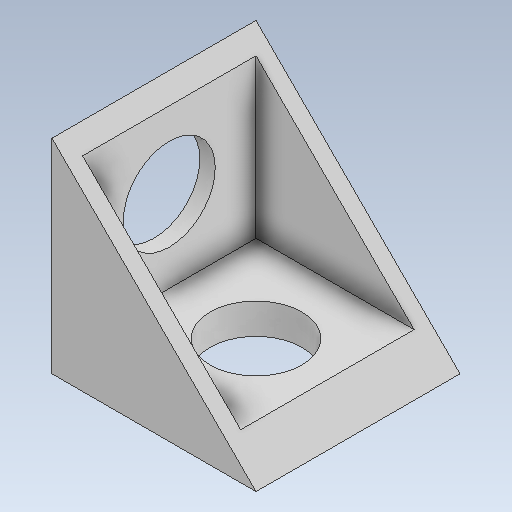
# Autodesk Inventor part: corner bracket
Saved by Autodesk Inventor 2023 (Build 270158000, 158)
## iProperties
Created: 2023-01-21
Part Number: corner bracket
Material: Generic
Document SubType Name: Modeling
Designer: eplym
Density: 1 g/cm^3
Appearance: Default
Author: eplym
Autodesk Inventor part; units mm, degrees
ref_plane "YZ Plane" through (0, 0, 0) normal (1, 0, 0) x (0, 1, 0)
ref_plane "XZ Plane" through (0, 0, 0) normal (0, 1, 0) x (-1, 0, 0)
ref_plane "XY Plane" through (0, 0, 0) normal (0, 0, 1) x (1, 0, 0)
sketch "Sketch1" plane through (0, 0, 0) normal (0, 1, 0) x (-1, 0, 0)
  line L0 (-10, 10) -> (10, 10)
  line L1 (10, 10) -> (10, -10)
  line L2 (10, -10) -> (-10, -10)
  line L3 (-10, -10) -> (-10, 10)
  line L4 (-10, 10) -> (10, -10) construction
  line L5 (10, 10) -> (-10, -10) construction
  point P0 (0, 0)
  dimension "d0" = 20
  dimension "d1" = 20
  constraints: 12 end point, 2 midpoint, 2 parallel, 1 horizontal, 1 perpendicular
  measures "d0" distance of L0.end L1.end
  measures "d1" distance of L1.end L2.end
extrude "Extrusion1" add sketch "Sketch1" along normal blind 20
sketch "Sketch2" plane through (0, 20, 0) normal (0, 1, 0) x (1, 0, 0)
  line L0 (8.5, -8.5) -> (-8.5, -8.5)
  line L1 (-8.5, -8.5) -> (-8.5, 8.5)
  line L2 (-8.5, 8.5) -> (8.5, 8.5)
  line L3 (8.5, 8.5) -> (8.5, -8.5)
  line L4 (8.5, -8.5) -> (-8.5, 8.5) construction
  line L5 (-8.5, -8.5) -> (8.5, 8.5) construction
  point P0 (0, 0)
  dimension "d4" = 17
  dimension "d5" = 17
  constraints: 12 end point, 2 midpoint, 2 parallel, 1 horizontal, 1 perpendicular
  measures "d4" distance of L0.end L1.end
  measures "d5" distance of L1.end L2.end
extrude "Extrusion2" cut sketch "Sketch2" against normal blind 17
sketch "Sketch6" plane through (-10, 0, 10) normal (0, 0, 1) x (1, 0, 0)
  line L0 (20, 0) -> (0, 0) projected
  line L1 (0, 20) -> (20, 0)
  line L2 (20, 0) -> (20, 20)
  line L3 (20, 20) -> (0, 20)
  line L4 (1.5, 20) -> (18.5, 20) projected
  point P0 (10, 0)
  constraints: 6 end point, 1 collinear, 1 perpendicular
extrude "Extrusion6" cut sketch "Sketch6" against normal through all
sketch "Sketch7" plane through (0, 3, 0) normal (0, 1, 0) x (1, 0, 0)
  circle A0 centre (0, 0) radius 4.5
  dimension "d20" = 9
  constraints: 1 centre point, 1 coincident
  measures "d20" diameter of A0
sketch "Sketch8" plane through (-8.5, 3, 8.5) normal (1, 0, 0) x (0, 0, -1)
  circle A0 centre (8.5, 8) radius 4.5
  line L0 (0, 0) -> (17, 0) projected
  point P0 (8.5, -3)
  dimension "d18" = 8
  dimension "d19" = 9
  constraints: 1 centre point
  measures "d18" distance from line of L0 A0.centre
  measures "d19" diameter of A0
extrude "Extrusion7" cut sketch "Sketch8" against normal blind 10
extrude "Extrusion8" cut sketch "Sketch7" against normal blind 10
body "Solid1"
